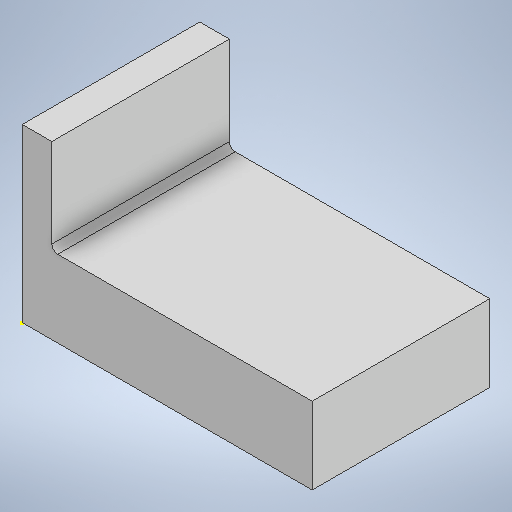
# Autodesk Inventor part: small_microswitch_holder
Saved by Autodesk Inventor 2025.2 (Build 292293000, 293)
## iProperties
Created: 2025-04-01
Part Number: small_microswitch_holder
Material: Generic
Document SubType Name: Modeling
Designer: osmon
Density: 1 g/cm^3
Appearance: Default
Author: osmon
Autodesk Inventor part; units mm, degrees
ref_plane "YZ Plane" through (0, 0, 0) normal (1, 0, 0) x (0, 1, 0)
ref_plane "XZ Plane" through (0, 0, 0) normal (0, 1, 0) x (-1, 0, 0)
ref_plane "XY Plane" through (0, 0, 0) normal (0, 0, 1) x (1, 0, 0)
sketch "Sketch1" plane through (0, 0, 0) normal (0, 1, 0) x (-1, 0, 0)
  point P0 (0, 0)
sketch "Sketch2" plane through (0, 0, 0) normal (0, 1, 0) x (-1, 0, 0)
  line L0 (0, 0) -> (-24.5, 0)
  line L1 (-24.5, 0) -> (-24.5, -15)
  line L2 (-24.5, -15) -> (0, -15)
  line L3 (0, -15) -> (0, 0)
  dimension "d0" = 24.5
  dimension "d1" = 15
  constraints: 8 end point, 2 parallel, 1 horizontal, 1 perpendicular
  measures "d0" distance of L2.end L1.end
  measures "d1" distance of L1.end L0.end
extrude "Extrusion1" add sketch "Sketch2" along normal blind 6.5
sketch "Sketch3" plane through (0, 6.5, 0) normal (0, 1, 0) x (1, 0, 0)
  line L0 (0, 15) -> (0, 0) projected
  line L1 (24.5, 15) -> (0, 15) projected
  line L2 (0, 0) -> (2.5, 0)
  line L3 (2.5, 0) -> (2.5, 15)
  line L4 (2.5, 15) -> (0, 15)
  line L5 (0, 15) -> (0, 0)
  dimension "d4" = 2.5
  constraints: 8 end point, 2 parallel, 1 horizontal, 1 perpendicular, 1 point on line
  measures "d4" distance of L4.end L3.end
extrude "Extrusion2" add sketch "Sketch3" along normal blind 8
fillet "Fillet1" radius 0.5 1 edges at (2.5, 6.5, -7.5)
body "Solid1"
